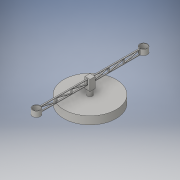
# Autodesk Inventor part: Centre structure
Saved by Autodesk Inventor 2016 SP1 (Build 200210100, 210)
## iProperties
Created: 2016-02-19
Part Number: Centre structure
Material: Generic
Document SubType Name: Modeling
Designer: Tore Den Store
Density: 1 g/cm^3
Appearance: Default
Author: Tore Den Store
Autodesk Inventor part; units mm, degrees
ref_plane "YZ Plane" through (0, 0, 0) normal (1, 0, 0) x (0, 1, 0)
ref_plane "XZ Plane" through (0, 0, 0) normal (0, 1, 0) x (-1, 0, 0)
ref_plane "XY Plane" through (0, 0, 0) normal (0, 0, 1) x (1, 0, 0)
sketch "Sketch1" plane through (0, 0, 0) normal (0, 0, 1) x (1, 0, 0)
  circle A0 centre (0, 0) radius 1000
  dimension "d0" = 2000
  constraints: 1 centre point, 1 coincident
  measures "d0" diameter of A0
extrude "Extrusion1" add sketch "Sketch1" against normal blind 300
sketch "Sketch2" plane through (0, 0, -300) normal (0, 0, -1) x (-1, 0, 0)
  circle A0 centre (0, 0) radius 1000 projected
  circle A1 centre (0, 0) radius 100
  dimension "d3" = 200
  constraints: 1 centre point, 1 coincident
  measures "d3" diameter of A1
extrude "Extrusion2" add sketch "Sketch2" along normal blind 200 contours A1
sketch "Sketch3" plane through (0, 0, -500) normal (0, 0, -1) x (-1, 0, 0)
  line L0 (-100, 100) -> (100, 100)
  line L1 (100, 100) -> (100, -100)
  line L2 (100, -100) -> (-100, -100)
  line L3 (-100, -100) -> (-100, 100)
  line L4 (-100, 100) -> (100, -100) construction
  line L5 (100, 100) -> (-100, -100) construction
  point P0 (0, 0)
  dimension "d6" = 200
  dimension "d7" = 200
  constraints: 12 end point, 2 midpoint, 2 parallel, 1 horizontal, 1 perpendicular
  measures "d6" distance between parallel lines of L0 L2
  measures "d7" distance between parallel lines of L3 L1
extrude "Extrusion3" add sketch "Sketch3" along normal blind 400
sketch "Sketch4" plane through (0, 100, -500) normal (0, 1, 0) x (1, 0, 0)
  line L0 (-100, 400) -> (100, 400) projected
  line L1 (100, 0) -> (100, 400) projected
  line L2 (-20, 370) -> (20, 370)
  line L3 (20, 370) -> (20, 170)
  line L4 (20, 170) -> (-20, 170)
  line L5 (-20, 170) -> (-20, 370)
  point P0 (0, -500)
  dimension "d22" = 40
  dimension "d23" = 200
  dimension "d24" = 80
  dimension "d25" = 30
  constraints: 8 end point, 2 parallel, 1 horizontal, 1 perpendicular
  measures "d22" distance of L3.end L4.end
  measures "d23" distance of L2.end L3.end
  measures "d24" distance between parallel lines of L1 L3
  measures "d25" distance between parallel lines of L0 L2
extrude "Extrusion4" add sketch "Sketch4" along normal blind 1800
sketch "Sketch6" plane through (-20, 100, -670) normal (0, 0, 1) x (1, 0, 0)
  circle A0 centre (20, 1948.6607) radius 150
  circle A1 centre (20, 1948.6607) radius 130
  line L0 (40, 1800) -> (0, 1800) projected
  line L1 (0, 0) -> (0, 1800) projected
  line L2 (40, 0) -> (40, 1800) projected
  point P0 (0, -100)
  dimension "d18" = 300
  dimension "d19" = 20
  constraints: 2 centre point, 2 point on circle
  measures "d18" diameter of A0
  measures "d19" radial gap between concentric circles of A0 A1
extrude "Extrusion7" add sketch "Sketch6" against normal blind 210 contours A0 L0 picked at (18.6655, 1806.2408)
sketch "Sketch8" plane through (20, 100, -670) normal (1, 0, 0) x (0, 0, -1)
  line L0 (200, 0) -> (200, 1800) projected
  line L1 (200, 1800) -> (0, 1800) projected
  line L2 (0, 0) -> (0, 1800) projected
  line L3 (180, 1780) -> (20, 1780)
  line L4 (20, 1780) -> (20, 20)
  line L5 (20, 20) -> (180, 20)
  line L6 (180, 20) -> (180, 1780)
  line L7 (0, 0) -> (200, 0) projected
  point P0 (-670, -100)
  dimension "d32" = 20
  dimension "d33" = 20
  dimension "d34" = 20
  dimension "d35" = 20
  constraints: 8 end point, 2 parallel, 1 horizontal, 1 perpendicular
  measures "d32" distance between parallel lines of L0 L6
  measures "d33" distance between parallel lines of L3 L1
  measures "d34" distance between parallel lines of L2 L4
  measures "d35" distance between parallel lines of L7 L5
extrude "Extrusion8" cut sketch "Sketch8" against normal up to next contours L6 L5 L4 L3
sketch "Sketch11" plane through (20, 100, -670) normal (1, 0, 0) x (0, 0, -1)
  line L0 (180, 1780) -> (180, 20) projected
  line L1 (20, 1780) -> (180, 1780) projected
  line L2 (20, 20) -> (20, 1780) projected
  line L3 (180, 20) -> (20, 20) projected
  line L4 (180, 1200) -> (20, 1200)
  line L5 (20, 1180) -> (180, 1180)
  line L6 (180, 620) -> (20, 620)
  line L7 (20, 600) -> (180, 600)
  line L8 (180, 1780) -> (20, 1780) projected
  line L9 (180, 1180) -> (35, 620)
  line L10 (20, 620) -> (165, 1180)
  line L11 (180, 600) -> (35, 20)
  line L12 (165, 600) -> (20, 20)
  point P0 (-670, -100)
  dimension "d56" = 580
  dimension "d57" = 20
  dimension "d58" = 20
  dimension "d59" = 580
  dimension "d61" = 15
  dimension "d62" = 15
  dimension "d63" = 15
  constraints: 16 end point, 12 point on line, 4 perpendicular, 1 parallel
  measures "d56" distance between parallel lines of L1 L4
  measures "d57" distance between parallel lines of L5 L4
  measures "d58" distance between parallel lines of L7 L6
  measures "d59" distance between parallel lines of L3 L7
  measures "d61" distance of L10.end L5.end
  measures "d62" distance of L6.end L9.end
  measures "d63" distance of L12.start L7.end
extrude "Extrusion11" add sketch "Sketch11" against normal up to surface (40 mm away) contours L0 L5 L2 L4 | L9 L6 L10 L5 | L0 L7 L2 L6 | L11 L3 L12 L7
sketch "Sketch12" plane through (20, 100, -670) normal (1, 0, 0) x (0, 0, -1)
  line L0 (180, 1780) -> (180, 1200) projected
  line L1 (20, 1780) -> (180, 1780) projected
  line L2 (20, 1200) -> (20, 1780) projected
  line L3 (180, 1200) -> (20, 1200) projected
  line L4 (180, 1780) -> (35, 1200)
  line L5 (20, 1200) -> (165, 1780)
  point P0 (-670, -100)
  dimension "d66" = 15
  constraints: 4 end point, 2 point on line, 1 parallel
  measures "d66" distance of L5.end L0.start
extrude "Extrusion12" add sketch "Sketch12" against normal up to surface (40 mm away) contours L4 L3 L5 L1
mirror "Mirror1" about plane through (0, 0, 0) normal (0, 1, 0) of "Extrusion4", "Extrusion7", "Extrusion12", "Extrusion11", "Extrusion8"
equation "\"d58\" = d57"
equation "\"d63\" = d62"
body "Solid1"
